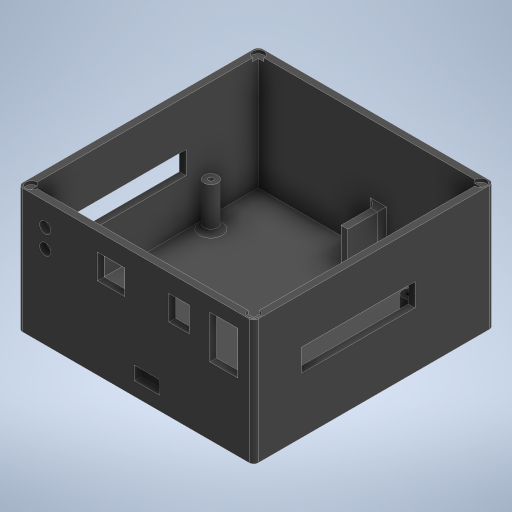
# Autodesk Inventor part: Base Chassis
Saved by Autodesk Inventor 2023 (Build 270158000, 158)
## iProperties
Created: 2023-03-17
Part Number: Base Chassis
Material: Generic
Document SubType Name: Modeling
Designer: Ahmed Nazir
Density: 1 g/cm^3
Appearance: Default
Author: Ahmed Nazir
Autodesk Inventor part; units mm, degrees
ref_plane "YZ Plane" through (0, 0, 0) normal (1, 0, 0) x (0, 1, 0)
ref_plane "XZ Plane" through (0, 0, 0) normal (0, 1, 0) x (-1, 0, 0)
ref_plane "XY Plane" through (0, 0, 0) normal (0, 0, 1) x (1, 0, 0)
sketch "Sketch1" plane through (0, 0, 0) normal (0, 1, 0) x (-1, 0, 0)
  line L0 (0, 0) -> (-98, 0)
  line L1 (-98, 0) -> (-98, -100)
  line L2 (-98, -100) -> (0, -100)
  line L3 (0, -100) -> (0, 0)
  line L4 (3, -103) -> (-101, -103)
  line L5 (-101, -103) -> (-101, 3)
  line L6 (-101, 3) -> (3, 3)
  line L7 (3, 3) -> (3, -103)
  line L8 (0, -20) -> (-6, -20)
  line L9 (-6, -20) -> (-6, -80)
  line L10 (-6, -80) -> (0, -80)
  line L11 (0, -80) -> (0, -20)
  line L12 (-46, -20) -> (-52, -20)
  line L13 (-52, -20) -> (-52, -80)
  line L14 (-52, -80) -> (-46, -80)
  line L15 (-46, -80) -> (-46, -20)
  line L16 (-92, -20) -> (-98, -20)
  line L17 (-98, -20) -> (-98, -80)
  line L18 (-98, -80) -> (-92, -80)
  line L19 (-92, -80) -> (-92, -20)
  point P0 (-49, -20)
  point P1 (-6, -50)
  point P2 (-98, -20)
  point P3 (-98, -80)
  point P4 (0, -80)
  point P5 (0, -20)
  dimension "d0" = 100
  dimension "d1" = 98
  dimension "d2" = 3
  dimension "d48" = 6
  dimension "d49" = 60
  dimension "d50" = 6
  dimension "d51" = 60
  dimension "d52" = 6
  dimension "d53" = 60
  dimension "d54" = 49
  dimension "d55" = 50
  constraints: 40 end point, 10 parallel, 5 perpendicular, 4 horizontal, 2 collinear, 2 midpoint, 2 point on line, 3 other
  measures "d0" distance of L1.end L0.end
  measures "d1" distance of L1.end L2.end
  measures "d2" distance between parallel lines of L2 L4
  measures "d48" distance of L10.end L9.end
  measures "d49" distance of L9.end L8.end
  measures "d50" distance of L14.end L13.end
  measures "d51" distance of L13.end L12.end
  measures "d52" distance of L18.end L17.end
  measures "d53" distance of L17.end L16.end
  measures "d54" distance from line of L1 point (-49, -20)
  measures "d55" distance from line of L0 point (-6, -50)
extrude "Extrusion1" add sketch "Sketch1" along normal blind 4 contours L3 L8 L9 L10 L2 L1 L18 L19 L16 L0 | L3 L10 L9 L8 | L16 L19 L18 L1 | L15 L14 L13 L12
extrude "Extrusion2" add sketch "Sketch1" along normal blind 55 contours L4 L5 L6 L7
fillet "Fillet1" radius 2 4 edges at (-3, 27.5, 3) (101, 27.5, 3) (101, 27.5, -103) (-3, 27.5, -103)
sketch "Sketch2" plane through (0, 4, 0) normal (0, 1, 0) x (1, 0, 0)
  line L0 (98, 0) -> (98, 100) projected
  line L1 (98, 100) -> (0, 100) projected
  line L2 (0, 100) -> (0, 0) projected
  line L3 (0, 0) -> (98, 0) projected
  circle A0 centre (5.185, 73.913) radius 3
  circle A1 centre (5.185, 6.858) radius 3
  circle A2 centre (92.815, 6.858) radius 3
  circle A3 centre (92.815, 73.913) radius 3
  line L4 (54.5, 100) -> (51.5, 100)
  line L5 (51.5, 100) -> (51.5, 85)
  line L6 (51.5, 85) -> (54.5, 85)
  line L7 (54.5, 85) -> (54.5, 100)
  line L8 (0, 100) -> (98, 100) projected
  dimension "d8" = 6
  dimension "d9" = 6
  dimension "d10" = 6
  dimension "d11" = 6
  dimension "d12" = 67.055
  dimension "d13" = 87.63
  dimension "d16" = 6.858
  dimension "d17" = 5.185
  dimension "d120" = 3
  dimension "d121" = 15
  dimension "d122" = 51.5
  constraints: 8 end point, 4 centre point, 2 horizontal alignment, 2 parallel, 2 vertical alignment, 1 collinear, 1 horizontal, 1 perpendicular
  measures "d8" diameter of A0
  measures "d9" diameter of A1
  measures "d10" diameter of A2
  measures "d11" diameter of A3
  measures "d12" distance of A1.centre A0.centre
  measures "d13" distance of A3.centre A0.centre
  measures "d16" distance from line of L3 A1.centre
  measures "d17" distance from line of L2 A1.centre
  measures "d120" distance of L6.end L5.end
  measures "d121" distance of L5.end L4.end
  measures "d122" distance between parallel lines of L5 L2
extrude "Extrusion3" add sketch "Sketch2" along normal blind 19 contours L7 L6 L5 L1 | A0 | A1 | A2 | A3
sketch "Sketch3" plane through (92.815, 23, -73.913) normal (0, 1, 0) x (1, 0, 0)
  circle A0 centre (0, -67.055) radius 3 projected
  circle A1 centre (0, -67.055) radius 1.05
  circle A2 centre (0, 0) radius 3 projected
  circle A3 centre (0, 0) radius 1.05
  circle A4 centre (-87.63, 0) radius 3 projected
  circle A5 centre (-87.63, 0) radius 1.05
  circle A6 centre (-87.63, -67.055) radius 3 projected
  circle A7 centre (-87.63, -67.055) radius 1.05
  point P0 (-92.815, -73.913)
  dimension "d21" = 2.1
  dimension "d22" = 2.1
  dimension "d23" = 2.1
  dimension "d24" = 2.1
  constraints: 4 centre point, 4 coincident
  measures "d21" diameter of A1
  measures "d22" diameter of A3
  measures "d23" diameter of A5
  measures "d24" diameter of A7
extrude "Extrusion4" cut sketch "Sketch3" against normal blind 5 contours A1 | A3 | A5 | A7
fillet "Fillet2" radius 2 4 edges at (89.815, 4, -73.913) (89.815, 4, -6.858) (2.185, 4, -6.858) (2.185, 4, -73.913)
extrude "Extrusion5" cut sketch "Sketch1" along normal blind 2 contours L3 L10 L9 L8 | L16 L19 L18 L1 | L15 L14 L13 L12
sketch "Sketch4" plane through (-1, 0, 3) normal (0, 0, 1) x (1, 0, 0)
  line L0 (11.185, 4) -> (1.185, 4) projected
  line L1 (98.815, 4) -> (88.815, 4) projected
  line L2 (99, 4) -> (55.5, 4) projected
  line L3 (1, 4) -> (99, 4) projected
  line L4 (98.815, 4) -> (88.815, 4) projected
  line L5 (11.185, 4) -> (1.185, 4) projected
  line L6 (1, 4) -> (1, 55) projected
  line L7 (1, 4) -> (1, 55) projected
  line L8 (99, 4) -> (99, 55) projected
  line L9 (99, 4) -> (99, 55) projected
  line L10 (45.1, 47) -> (33, 47)
  line L11 (33, 47) -> (33, 36)
  line L12 (33, 36) -> (45.1, 36)
  line L13 (45.1, 36) -> (45.1, 47)
  line L14 (49.315, 6) -> (60.315, 6)
  line L15 (60.315, 6) -> (60.315, 12)
  line L16 (60.315, 12) -> (49.315, 12)
  line L17 (49.315, 12) -> (49.315, 6)
  line L18 (64.5, 47) -> (73.5, 47)
  line L19 (73.5, 47) -> (73.5, 36)
  line L20 (73.5, 36) -> (64.5, 36)
  line L21 (64.5, 36) -> (64.5, 47)
  line L22 (9.185, 23) -> (3.185, 23) projected
  line L23 (96.815, 23) -> (90.815, 23) projected
  circle A0 centre (10.0225, 36.5908) radius 2.5
  circle A1 centre (10.0225, 44.8769) radius 2.5
  line L24 (82.6763, 48.8494) -> (94.9263, 48.8494)
  line L25 (94.9263, 48.8494) -> (94.9263, 29.8494)
  line L26 (94.9263, 29.8494) -> (82.6763, 29.8494)
  line L27 (82.6763, 29.8494) -> (82.6763, 48.8494)
  line L28 (82.6763, 48.8494) -> (94.9263, 29.8494) construction
  line L29 (94.9263, 48.8494) -> (82.6763, 29.8494) construction
  line L30 (0, 0) -> (100, 0) projected
  line L31 (55.5, 4) -> (52.5, 4) projected
  line L32 (52.5, 4) -> (1, 4) projected
  point P0 (1, 0)
  point P1 (69, 36)
  point P2 (73.5, 41.5)
  point P3 (60.315, 9)
  point P4 (49.315, 9)
  point P5 (54.815, 6)
  point P6 (54.815, 12)
  point P7 (6.185, 23)
  point P8 (39.05, 36)
  point P9 (93.815, 23)
  point P10 (88.8013, 39.3494)
  dimension "d56" = 11
  dimension "d57" = 19.4
  dimension "d59" = 12.1
  dimension "d60" = 11
  dimension "d61" = 9
  dimension "d62" = 11
  dimension "d63" = 6
  dimension "d106" = 39
  dimension "d108" = 5
  dimension "d109" = 5
  dimension "d111" = 12.25
  dimension "d112" = 19
  dimension "d117" = 32
  dimension "d118" = 47
  dimension "d119" = 12
  constraints: 36 end point, 11 midpoint, 8 parallel, 4 horizontal, 4 perpendicular, 2 centre point, 1 collinear, 1 vertical alignment
  measures "d56" distance between parallel lines of L12 L10
  measures "d57" distance between parallel lines of L21 L13
  measures "d59" distance of L10.start L10.end
  measures "d60" distance from line of point (69, 36) L18
  measures "d61" distance from line of point (73.5, 41.5) L21
  measures "d62" distance of point (60.315, 9) point (49.315, 9)
  measures "d63" distance of point (54.815, 6) point (54.815, 12)
  measures "d106" horizontal distance of point (93.815, 23) point (54.815, 12)
  measures "d108" diameter of A0
  measures "d109" diameter of A1
  measures "d111" distance of L25.end L26.end
  measures "d112" distance of L24.end L25.end
  measures "d117" distance between parallel lines of L11 L7
  measures "d118" distance between parallel lines of L30 L10
  measures "d119" distance between parallel lines of L30 L16
extrude "Extrusion6" cut sketch "Sketch4" against normal up to surface (3 mm away)
sketch "Sketch5" plane through (101, 0, 1) normal (1, 0, 0) x (0, 0, -1)
  line L0 (12.858, 4) -> (2.858, 4) projected
  line L1 (79.913, 4) -> (69.913, 4) projected
  line L2 (1, 4) -> (101, 4) projected
  line L3 (101, 4) -> (1, 4) projected
  line L4 (12.858, 4) -> (2.858, 4) projected
  line L5 (79.913, 4) -> (69.913, 4) projected
  line L6 (1, 36) -> (1, 47) projected
  line L7 (1, 47) -> (1, 36) projected
  line L8 (1, 47) -> (1, 36) projected
  line L9 (1, 36) -> (1, 47) projected
  line L10 (1, 4) -> (1, 55) projected
  line L11 (1, 4) -> (1, 55) projected
  line L12 (10.858, 23) -> (4.858, 23) projected
  line L13 (77.913, 23) -> (71.913, 23) projected
  line L14 (19.133, 24.6) -> (69.133, 24.6)
  line L15 (69.133, 24.6) -> (69.133, 34.6)
  line L16 (69.133, 34.6) -> (19.133, 34.6)
  line L17 (19.133, 34.6) -> (19.133, 24.6)
  line L18 (12.858, 4) -> (2.858, 4) projected
  line L19 (4.858, 6) -> (10.858, 6) projected
  line L20 (79.913, 4) -> (69.913, 4) projected
  line L21 (71.913, 6) -> (77.913, 6) projected
  line L22 (1, 12) -> (1, 6) projected
  line L23 (1, 6) -> (1, 12) projected
  line L24 (101, 4) -> (86, 4) projected
  line L25 (86, 4) -> (101, 4) projected
  point P0 (1, 0)
  point P1 (74.913, 23)
  dimension "d1" = 98
  dimension "d98" = 10
  dimension "d99" = 50
  dimension "d101" = 1.6
  dimension "d102" = 5.78
  constraints: 8 end point, 2 parallel, 1 horizontal, 1 midpoint, 1 perpendicular
  measures "d98" distance between parallel lines of L14 L16
  measures "d99" distance of L15.end L16.end
  measures "d101" distance between parallel lines of L13 L14
  measures "d102" distance from line of point (74.913, 23) L15
sketch "Sketch6" plane through (-3, 0, -101) normal (-1, 0, 0) x (0, 0, 1)
  line L0 (32.867, 34.6) -> (82.867, 34.6) projected
  line L1 (32.867, 24.6) -> (32.867, 34.6) projected
  line L2 (82.867, 24.6) -> (32.867, 24.6) projected
  line L3 (82.867, 34.6) -> (82.867, 24.6) projected
  point P0 (101, 0)
extrude "Extrusion7" cut sketch "Sketch5" against normal up to surface (3 mm away)
extrude "Extrusion8" cut sketch "Sketch6" against normal up to surface (3 mm away)
sketch "Sketch7" plane through (0, 55, 0) normal (0, 1, 0) x (1, 0, 0)
  circle A0 centre (0, 100) radius 2.5
  circle A1 centre (0, 0) radius 2.5
  line L0 (98, 100) -> (98, 0) projected
  circle A2 centre (98, 100) radius 2.5
  circle A3 centre (98, 0) radius 2.5
  dimension "d113" = 5
  dimension "d114" = 5
  dimension "d115" = 5
  dimension "d116" = 5
  constraints: 4 centre point, 1 coincident
  measures "d113" diameter of A0
  measures "d114" diameter of A1
  measures "d115" diameter of A2
  measures "d116" diameter of A3
extrude "Extrusion9" cut sketch "Sketch7" against normal blind 1.5
fillet "Fillet3" radius 2 6 edges at (51.5, 4, -92.5) (53, 4, -85) (54.5, 4, -92.5) (54.5, 13.5, -100) (51.5, 13.5, -100) (53, 23, -100)
equation "\"d54\" = 0.5 * d1"
equation "\"d55\" = 0.5 * d0"
equation "\"d60\" = d56"
body "Solid1"
